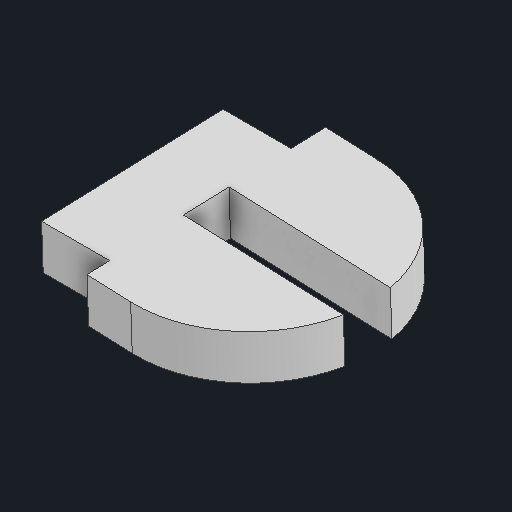
# Autodesk Inventor part: sponson_spanner_side_holder
Saved by Autodesk Inventor 2023 (Build 270158030, 158C)
## iProperties
Created: 2022-03-22
Part Number: sponson_spanner_side_holder
Material: Generic
Document SubType Name: Modeling
Designer: kardo
Density: 1 g/cm^3
Appearance: Default
Author: kardo
Autodesk Inventor part; units mm, degrees
ref_plane "YZ Plane" through (0, 0, 0) normal (1, 0, 0) x (0, 1, 0)
ref_plane "XZ Plane" through (0, 0, 0) normal (0, 1, 0) x (-1, 0, 0)
ref_plane "XY Plane" through (0, 0, 0) normal (0, 0, 1) x (1, 0, 0)
derived "parameters_frame.ipt"
derived "surface_body.ipt"
ref_plane "plane_tunnel_right" through (81.12, 0, 0) normal (1, 0, 0) x (0, 1, 0)
ref_plane "plane_sponson_side" through (81.12, 237, 36.448) normal (0.0378267, 0.0348745, -0.9986756) x (0.3011979, -0.9533106, -0.0218819)
derived "stencil_frame.ipt"
sketch "sk_joint_locations" plane through (81.12, 0, 0) normal (1, 0, 0) x (0, 1, 0)
  line L0 (0, 0) -> (122.4, 8.559) construction
  line L1 (36.465, 28.832) -> (112.2, 28.832) construction
  arc A0 (36.465, 28.832) -> (11.22, 28.376) centre (36.465, -670.197) ccw construction
  line L2 (-241.5001, 19.2432) -> (11.22, 28.376) construction
  line L3 (-345, 16.32) -> (-262.2001, 18.586) construction
  arc A1 (-262.2001, 18.586) -> (-241.5001, 19.2432) centre (-326.8578, 2381.2399) ccw construction
  line L4 (-95.1358, 3119.4657) -> (254.2444, -1876.9042) construction
  line L5 (-230.0001, 3089.1136) -> (-230.0001, -1866.0023) construction
  line L6 (-114.9999, 3089.1136) -> (-114.9999, -1866.0023) construction
  line L7 (-345, 3089.1136) -> (-345, -1866.0023) construction
  line L8 (0, 3089.1136) -> (0, -1866.0023) construction
  line L9 (516.4305, 45.5774) -> (-594.5903, 6.7797) construction
  line L10 (-657.7604, -27.3784) -> (621.8174, 62.0984) construction
  line L11 (193.4506, 30.2962) -> (193.1714, 38.2913) construction
  line L12 (201.1621, 36.7028) -> (201.7215, 28.7028) construction
  line L13 (0, 14.96) -> (121.9304, 15.2746) construction
  line L14 (-230.0001, 45.8702) -> (-230.0001, 19.6588) construction
  line L15 (-345, 37.4554) -> (-345, 16.32) construction
  line L16 (-114.9999, 51.0173) -> (-114.9999, 23.8147) construction
  line L17 (0, 52.89) -> (0, 27.9705) construction
  line L18 (119.462, 50.575) -> (119.9556, 43.5149) construction
  line L19 (120.4493, 36.4549) -> (119.9556, 43.5149) construction
  line L20 (120.4493, 36.4549) -> (120.943, 29.3948) construction
  line L21 (120.943, 29.3948) -> (121.4367, 22.3347) construction
  line L22 (121.4367, 22.3347) -> (121.9304, 15.2746) construction
  line L23 (0, 14.96) -> (0, 0) construction
  line L24 (112.2, 37.536) -> (112.2, 28.832) construction
  line L25 (112.2, 35.548) -> (112.2, 30.82) construction
  spline S0 degree 4 poles (-345, 37.4554) (-258.8682, 45.1562) (-172.5926, 49.7838) (-86.3161, 52.89) (0, 52.89) knots 0 0 0 0 0 1 1 1 1 1
  spline S1 degree 3 poles (0, 52.89) (92.8353, 52.89) (195.0311, 49.5089) (255, 36.448) knots 0 0 0 0 1 1 1 1
  spline S2 degree 2 poles (122.4, 8.559) (190.3044, 13.3074) (255, 36.448) knots 0 0 0 1 1 1
  point P0 (-95.1358, 3119.4657)
  point P1 (254.2444, -1876.9042)
  point P2 (193.311, 34.2938)
  point P3 (201.4418, 32.7028)
  point P4 (134.9575, 11.3411)
  point P5 (-345, 26.8877)
  point P6 (-230.0001, 32.7645)
  point P7 (-114.9999, 37.416)
  point P8 (0, 40.4303)
  point P9 (112.2, 33.184)
ref_plane "plane_base" through (81.12, 193.311, 34.2938) normal (0, -0.9993908, -0.0348995) x (1, 0, 0)
sketch "sk_base" plane through (81.12, 193.311, 34.2938) normal (0, -0.9993908, -0.0348995) x (1, 0, 0)
  line L0 (0, 2978.5787) -> (0, -1320.4667) projected
  line L1 (141.5251, 5.9855) -> (-149.2681, -5.0222) construction
  line L2 (10.3907, -0.9799) -> (3, -1.2597)
  line L3 (3, -1.2597) -> (3, 0.7418)
  line L4 (3, 0.7418) -> (10.315, 1.0187)
  line L5 (0, 4) -> (3, 4)
  line L6 (3, 4) -> (3, 5)
  line L7 (3, 5) -> (4.9986, 5.0757)
  line L8 (0, -4) -> (3, -4)
  line L9 (3, -4) -> (3, -5.5179)
  line L10 (3, -5.5179) -> (5.3961, -5.4272)
  arc A0 (5.3961, -5.4272) -> (4.9986, 5.0757) centre (5.1974, -0.1758) ccw
  line L11 (3, -0.259) -> (10.4488, 0.023) construction
  line L12 (4.9986, 5.0757) -> (5.3961, -5.4272) construction
  point P0 (-81.12, -27.5264)
  dimension "d3" = 3
  dimension "d4" = 2
  dimension "d5" = 2
  dimension "d6" = 1
  constraints: 22 end point, 5 parallel, 5 point on circle, 3 collinear, 2 perpendicular, 2 tangent, 1 centre point, 1 midpoint, 1 point on line
  measures "d3" distance between parallel lines of L0 L6
  measures "d4" distance between parallel lines of L1 L2
  measures "d5" distance of L6.end L7.end
  measures "d6" distance of L5.end L6.end
extrude "thicken" add sketch "sk_base" along normal blind 2 contours L5 L6 L7 A0 L4 L3 L2 L10 L9 L8 L0
equation "\"d3\" = stringer_thickness"
equation "\"d4\" = bulkhead_thickness"
equation "\"d5\" = bulkhead_thickness"
equation "\"d6\" = 0.5 * bulkhead_thickness"
equation "\"d7\" = bulkhead_thickness"
equation "\"stringer_thickness\" = 3"
equation "\"bulkhead_thickness\" = 2"
body "Solid1"
